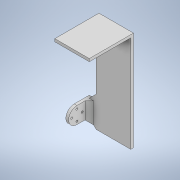
# Autodesk Inventor part: Part1
Saved by Autodesk Inventor 2020 (Build 240168000, 168)
## iProperties
Created: 2019-12-26
Part Number: Part1
Material: Generic
Document SubType Name: Modeling
Designer: tdmp4
Density: 1 g/cm^3
Appearance: Default
Author: tdmp4
Autodesk Inventor part; units mm, degrees
ref_plane "YZ Plane" through (0, 0, 0) normal (1, 0, 0) x (0, 1, 0)
ref_plane "XZ Plane" through (0, 0, 0) normal (0, 1, 0) x (-1, 0, 0)
ref_plane "XY Plane" through (0, 0, 0) normal (0, 0, 1) x (1, 0, 0)
sketch "Sketch1" plane through (0, 0, 0) normal (1, 0, 0) x (0, 1, 0)
  circle A0 centre (0, 0) radius 15.24
  circle A1 centre (9.779, 0) radius 1.7859
  circle A2 centre (0, -9.779) radius 1.7859
  circle A3 centre (-9.779, 0) radius 1.7859
  circle A4 centre (0, 9.779) radius 1.7859
  arc A5 (-1.7785, -9.6159) -> (1.7785, -9.6159) centre (0, 0) ccw
  dimension "d0" = 30.48
  dimension "d2" = 3.5719
  dimension "d3" = 3.5719
  dimension "d4" = 3.5719
  dimension "d5" = 3.5719
  constraints: 6 centre point, 5 point on circle, 2 coincident
  measures "d0" diameter of A0
  measures "d2" diameter of A1
  measures "d3" diameter of A2
  measures "d4" diameter of A3
  measures "d5" diameter of A4
extrude "Extrusion1" add sketch "Sketch1" along normal blind 5.08
sketch "Sketch5" plane through (5.08, 0, 0) normal (1, 0, 0) x (0, 0, -1)
  circle A0 centre (0, 0) radius 15.24 projected
  arc A1 (0, -15.24) -> (0, 15.24) centre (0, 0) ccw
  line L0 (0, 15.24) -> (27.94, 15.24)
  line L1 (27.94, 15.24) -> (27.94, -15.24)
  line L2 (27.94, -15.24) -> (0, -15.24)
  dimension "d17" = 27.94
  dimension "d18" = 30.48
  constraints: 6 end point, 4 point on circle, 2 tangent, 1 centre point, 1 horizontal, 1 perpendicular, 1 vertical
  measures "d17" distance of L0.start L0.end
  measures "d18" distance of L0.end L1.end
extrude "Extrusion3" add sketch "Sketch5" against normal blind 5.08 contours A0 L0 L1 L2
sketch "Sketch6" plane through (5.08, 0, 0) normal (1, 0, 0) x (0, 0, -1)
  line L0 (27.94, -15.24) -> (27.94, 15.24) projected
  line L1 (27.94, -15.24) -> (22.86, -15.24)
  line L2 (22.86, -15.24) -> (22.86, 15.6141)
  line L3 (22.86, 15.6141) -> (27.94, 15.6141)
  line L4 (27.94, 15.6141) -> (27.94, -15.24)
  point P0 (0, 0)
  dimension "d21" = 5.08
  constraints: 8 end point, 2 parallel, 1 horizontal, 1 perpendicular
  measures "d21" distance of L2.end L3.end
extrude "Extrusion4" add sketch "Sketch6" along normal blind 12.7
sketch "Sketch7" plane through (0, -15.24, -27.94) normal (0, 0, -1) x (-1, 0, 0)
  line L0 (-17.78, 30.8541) -> (-17.78, 0) projected
  line L1 (-17.78, 0) -> (-81.28, 0)
  line L2 (-81.28, 0) -> (-81.28, 165.1)
  line L3 (-81.28, 165.1) -> (-17.78, 165.1)
  line L4 (-17.78, 165.1) -> (-17.78, 0)
  line L5 (-5.08, 0) -> (-17.78, 0) projected
  line L6 (-17.78, 0) -> (-81.28, 0)
  line L7 (-81.28, 0) -> (-81.28, -12.7)
  line L8 (-81.28, -12.7) -> (-17.78, -12.7)
  line L9 (-17.78, -12.7) -> (-17.78, 0)
  point P0 (0, 15.24)
  dimension "d24" = 63.5
  dimension "d25" = 165.1
  dimension "d26" = 12.7
  constraints: 16 end point, 4 parallel, 2 horizontal, 2 perpendicular
  measures "d24" distance of L2.end L3.end
  measures "d25" distance of L1.end L2.end
  measures "d26" distance of L6.end L7.end
extrude "Extrusion5" add sketch "Sketch7" against normal blind 5.08
chamfer "Chamfer1" distance 7.9375 angle 45 1 edges at (5.08, 0, -22.86)
chamfer "Chamfer2" distance 12.7 angle 45 1 edges at (17.78, 15.6141, -25.4)
chamfer "Chamfer3" distance 12.7 angle 45 1 edges at (17.78, -15.24, -25.4)
sketch "Sketch9" plane through (0, -15.24, -27.94) normal (0, 0, -1) x (-1, 0, 0)
  line L0 (-23.8936, 160.265) -> (-30.2436, 160.265)
  line L1 (-30.2436, 160.265) -> (-30.2436, -9.915)
  line L2 (-30.2436, -9.915) -> (-23.8936, -9.915)
  line L3 (-23.8936, -9.915) -> (-23.8936, 160.265)
  line L4 (-48.0524, 160.265) -> (-54.4024, 160.265)
  line L5 (-54.4024, 160.265) -> (-54.4024, -9.915)
  line L6 (-54.4024, -9.915) -> (-48.0524, -9.915)
  line L7 (-48.0524, -9.915) -> (-48.0524, 160.265)
  line L8 (-65.8613, 160.265) -> (-72.2113, 160.265)
  line L9 (-72.2113, 160.265) -> (-72.2113, -9.915)
  line L10 (-72.2113, -9.915) -> (-65.8613, -9.915)
  line L11 (-65.8613, -9.915) -> (-65.8613, 160.265)
  line L12 (-20.035, 146.74) -> (-76.5781, 146.74)
  line L13 (-76.5781, 146.74) -> (-76.5781, 134.04)
  line L14 (-76.5781, 134.04) -> (-20.035, 134.04)
  line L15 (-20.035, 134.04) -> (-20.035, 146.74)
  line L16 (-3.4134, 23.4136) -> (-76.5781, 23.4136)
  line L17 (-76.5781, 23.4136) -> (-76.5781, 10.7136)
  line L18 (-76.5781, 10.7136) -> (-3.4134, 10.7136)
  line L19 (-3.4134, 10.7136) -> (-3.4134, 23.4136)
  point P0 (0, 15.24)
  point P1 (-30.2436, 134.04)
  point P2 (-30.2436, 23.4136)
  point P3 (-48.0524, 23.4136)
  point P4 (-48.0524, 134.04)
  point P5 (-54.4024, 134.04)
  point P6 (-54.4024, 23.4136)
  point P7 (-65.8613, 23.4136)
  point P8 (-65.8613, 134.04)
  point P9 (-30.2436, 146.74)
  point P10 (-48.0524, 146.74)
  point P11 (-54.4024, 146.74)
  point P12 (-65.8613, 146.74)
  point P13 (-72.2113, 146.74)
  point P14 (-72.2113, 134.04)
  point P15 (-72.2113, 23.4136)
  point P16 (-72.2113, 10.7136)
  point P17 (-65.8613, 10.7136)
  point P18 (-54.4024, 10.7136)
  point P19 (-48.0524, 10.7136)
  point P20 (-30.2436, 10.7136)
  point P21 (-23.8936, 10.7136)
  point P22 (-23.8936, 23.4136)
  point P23 (-23.8936, 134.04)
  point P24 (-23.8936, 146.74)
  dimension "d47" = 6.35
  dimension "d48" = 170.18
  dimension "d49" = 6.35
  dimension "d50" = 6.35
  dimension "d51" = 12.7
  dimension "d52" = 12.7
  constraints: 40 end point, 10 parallel, 5 horizontal, 5 perpendicular, 2 point on line
  measures "d47" distance of L2.end L1.end
  measures "d48" distance of L2.end L0.start
  measures "d49" distance of L6.end L5.end
  measures "d50" distance of L10.end L9.end
  measures "d51" distance of L12.end L13.end
  measures "d52" distance of L16.end L17.end
extrude "Extrusion6" add sketch "Sketch9" along normal blind 2.54 contours L3 L12 L1 L0 | L12 L15 L14 L3 | L3 L14 L1 L12 | L1 L14 L7 L12 | L3 L16 L1 L14 | L12 L5 L4 L7 | L7 L14 L5 L12 | L16 L19 L18 L3 | L3 L18 L1 L16 | L1 L18 L7 L16 | L7 L16 L5 L14 | L5 L14 L11 L12 | L3 L2 L1 L18 | L7 L18 L5 L16 | L12 L9 L8 L11 | L11 L14 L9 L12 | L7 L6 L5 L18 | L5 L18 L11 L16 | L11 L16 L9 L14 | L9 L14 L13 L12 | L11 L18 L9 L16 | L11 L10 L9 L18 | L9 L18 L17 L16
sketch "Sketch10" plane through (48.0524, 118.8, -27.94) normal (0, 0, -1) x (-1, 0, 0)
  line L0 (-33.2276, 31.06) -> (30.2724, 31.06)
  line L1 (30.2724, 31.06) -> (30.2724, 36.14)
  line L2 (30.2724, 36.14) -> (-33.2276, 36.14)
  line L3 (-33.2276, 36.14) -> (-33.2276, 31.06)
  point P0 (48.0524, -118.8)
  dimension "d55" = 63.5
  dimension "d56" = 5.08
  constraints: 8 end point, 2 parallel, 1 horizontal, 1 perpendicular
  measures "d55" distance of L2.end L1.end
  measures "d56" distance of L0.end L1.end
extrude "Extrusion7" add sketch "Sketch10" against normal blind 81.28
body "Solid1"
